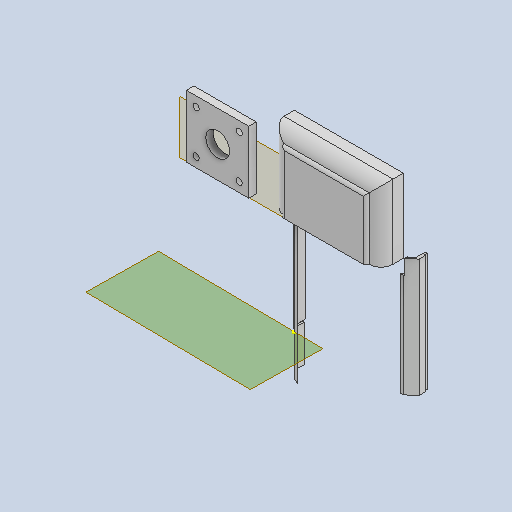
# Autodesk Inventor part: крышка камера
Saved by Autodesk Inventor 2024.2 (Build 282272000, 272)
## iProperties
Created: 2025-10-05
Part Number: крышка камера
Material: Типовые
Document SubType Name: Modeling
Designer: katya_notebook
Density: 1 g/cm^3
Appearance: По умолчанию
Author: katya_notebook
Autodesk Inventor part; units mm, degrees
ref_plane "YZ Plane" through (0, 0, 0) normal (1, 0, 0) x (0, 1, 0)
ref_plane "XZ Plane" through (0, 0, 0) normal (0, 1, 0) x (-1, 0, 0)
ref_plane "XY Plane" through (0, 0, 0) normal (0, 0, 1) x (1, 0, 0)
ref_plane "РабПлоскость1" through (0, 97.1605, 0) normal (0, 0, 1) x (-1, 0, 0)
sketch "Эскиз1" plane through (0, 97.1605, 0) normal (0, 0, 1) x (-1, 0, 0)
  line L0 (53.6991, 17.5343) -> (19.6991, 17.5343) projected
  line L1 (0, -26.68) -> (0, 17.5343)
  line L2 (0, 17.5343) -> (-73.3991, 17.5343)
  line L3 (-73.3991, -26.68) -> (-73.3991, 17.5343)
  line L4 (0, -26.68) -> (0, -32.1685)
  line L5 (-73.3991, -26.68) -> (-73.3991, -32.1685)
  line L6 (-73.3991, -32.1685) -> (0, -32.1685)
  line L7 (-73.3991, 110.6606) -> (-73.3991, 83.6606) projected
  constraints: 12 end point, 2 perpendicular, 1 horizontal, 1 vertical
extrude "Выдавливание1" add sketch "Эскиз1" along normal blind 15
sketch "Эскиз2" plane through (0, 97.1605, 0) normal (0, 0, -1) x (1, 0, 0)
  point P0 (0, 97.1605)
sketch "Эскиз3" plane through (0, 97.1605, 0) normal (0, 0, 1) x (-1, 0, 0)
  circle A0 centre (36.6991, -1.4657) radius 8 projected
  line L0 (53.6991, 17.5343) -> (19.6991, 17.5343) projected
  line L1 (19.6991, -20.4657) -> (53.6991, -20.4657) projected
  line L2 (17.6991, 15.5343) -> (17.6991, -18.4657) projected
  line L3 (55.6991, -18.4657) -> (55.6991, 15.5343) projected
  line L4 (57.6991, 19.5343) -> (15.6991, 19.5343)
  line L5 (15.6991, 19.5343) -> (15.6991, -22.4657)
  line L6 (15.6991, -22.4657) -> (57.6991, -22.4657)
  line L7 (57.6991, -22.4657) -> (57.6991, 19.5343)
  line L8 (57.6991, 19.5343) -> (15.6991, -22.4657) construction
  line L9 (15.6991, 19.5343) -> (57.6991, -22.4657) construction
  point P0 (0, 97.1605)
  dimension "d2" = 42
  dimension "d3" = 42
  constraints: 12 end point, 2 midpoint, 2 parallel, 1 horizontal, 1 perpendicular
  measures "d2" distance of L6.end L5.end
  measures "d3" distance of L4.start L6.end
extrude "Выдавливание2" cut sketch "Эскиз3" along normal blind 15
sketch "Эскиз4" plane through (36.6991, -1.4657, 15) normal (0, 0, 1) x (1, 0, 0)
  circle A0 centre (0, 0) radius 8
  point P0 (-36.6991, 1.4657)
  dimension "d8" = 16
  constraints: 1 centre point
  measures "d8" diameter of A0
extrude "Выдавливание3" cut sketch "Эскиз4" against normal blind 15
sketch "Эскиз5" plane through (0, 97.1605, 15) normal (0, 0, 1) x (-1, 0, 0)
  line L0 (15.6991, 19.5343) -> (57.6991, 19.5343) projected
  line L1 (15.6991, -22.4657) -> (15.6991, 19.5343) projected
  line L2 (15.6991, 19.5343) -> (57.6991, 19.5343)
  line L3 (57.6991, 19.5343) -> (57.6991, -22.4657)
  line L4 (57.6991, -22.4657) -> (15.6991, -22.4657)
  line L5 (15.6991, -22.4657) -> (15.6991, 19.5343)
  circle A0 centre (36.6991, -1.4657) radius 8 projected
  circle A1 centre (36.6991, -1.4657) radius 8
  point P0 (0, 97.1605)
  constraints: 8 end point, 2 parallel, 1 centre point, 1 coincident, 1 concentric, 1 horizontal, 1 perpendicular
extrude "Выдавливание4" add sketch "Эскиз5" against normal blind 5
sketch "Эскиз6" plane through (0, 97.1605, 15) normal (0, 0, 1) x (-1, 0, 0)
  circle A0 centre (4.8591, -20.5207) radius 1.7 projected
  circle A1 centre (68.6491, -20.5207) radius 1.7 projected
  point P0 (0, 97.1605)
extrude "Выдавливание5" cut sketch "Эскиз6" against normal blind 15
ref_plane "РабПлоскость2" through (-83.6534, 0, 27.511) normal (0, -1, 0) x (0.9999139, 0, 0.0131203)
sketch "Эскиз7" plane through (-83.6534, 0, 27.511) normal (0, -1, 0) x (0.9999139, 0, 0.0131203)
  line L0 (79.6013, -33.3861) -> (83.2852, -28.6062) projected
  line L1 (79.5461, -37.5999) -> (79.6013, -33.3861) projected
  line L2 (75.3464, -37.5448) -> (79.5461, -37.5999) projected
  line L3 (83.2852, -28.6062) -> (79.6013, -33.3861)
  line L4 (79.6013, -33.3861) -> (79.5461, -37.5999)
  line L5 (1622.9751, -57.8519) -> (79.5461, -37.5999)
  line L6 (1622.9751, -57.8519) -> (1622.9751, -55.8519)
  line L7 (1622.9751, -55.8519) -> (1621.8385, -55.8519)
  line L8 (1621.8385, -55.8519) -> (1619.8385, -55.8519)
  line L9 (83.2852, -28.6062) -> (85.2851, -28.6324)
  line L10 (156.6781, -29.5692) -> (83.2852, -28.6062) projected
  line L11 (80.8455, -31.8201) -> (80.8455, -55.8519)
  line L12 (80.8455, -55.8519) -> (1619.8385, -55.8519)
  line L13 (80.8455, -31.8201) -> (85.2851, -28.6324)
  line L14 (46.6, -4.8277) -> (46.6, -53.2548)
  line L15 (13.5987, -33.3861) -> (9.9148, -28.6062)
  line L16 (13.6539, -37.5999) -> (13.5987, -33.3861)
  line L17 (9.9148, -28.6062) -> (13.5987, -33.3861)
  line L18 (13.5987, -33.3861) -> (13.6539, -37.5999)
  line L19 (-1529.7751, -57.8519) -> (13.6539, -37.5999)
  line L20 (-1529.7751, -57.8519) -> (-1529.7751, -55.8519)
  line L21 (-1529.7751, -55.8519) -> (-1528.6385, -55.8519)
  line L22 (-1528.6385, -55.8519) -> (-1526.6385, -55.8519)
  line L23 (9.9148, -28.6062) -> (7.9149, -28.6324)
  line L24 (12.3545, -31.8201) -> (12.3545, -55.8519)
  line L25 (12.3545, -55.8519) -> (-1526.6385, -55.8519)
  line L26 (12.3545, -31.8201) -> (7.9149, -28.6324)
  point P0 (87.0301, -15.4429)
  point P1 (85.1096, -24.071)
  point P2 (-1456.642, -15.4429)
  point P3 (1470.5529, -55.8519)
  point P4 (80.8455, -37.617)
  dimension "d13" = 2
  dimension "d14" = 2
  dimension "d15" = 2
  dimension "d16" = 2
  constraints: 46 end point, 10 symmetric about line, 3 vertical, 2 collinear, 2 horizontal, 2 perpendicular, 2 point on line
  measures "d13" distance of L6.end L5.start
  measures "d14" distance of L8.end L7.end
  measures "d15" distance of L0.end L9.end
  measures "d16" distance of L11.start L0.start
ref_plane "РабПлоскость3" through (-3.0009, -24.18, -16.4278) normal (0.7071068, 0.7071068, 0) x (-0.7071068, 0.7071068, 0)
extrude "Выдавливание6" add sketch "Эскиз7" against normal up to surface contours L0 L9 L13 L11 L5 L1 surface through (-3.0009, -24.18, -16.4278) normal (0.7071068, 0.7071068, 0)
ref_plane "РабПлоскость4" through (-83.6534, 0, 27.511) normal (0, -1, 0) x (0.9999139, 0, 0.0131203)
sketch "Эскиз8" plane through (-83.6534, 0, 27.511) normal (0, -1, 0) x (0.9999139, 0, 0.0131203)
  line L0 (6.28, -18.2609) -> (9.8931, -27.6692)
  line L1 (9.8931, -27.6692) -> (11.8779, -27.6692)
  line L2 (156.6781, -29.5692) -> (83.2852, -28.6062) projected
  line L3 (6.28, -9.4429) -> (6.28, -18.2609)
  line L4 (12.3545, -31.8201) -> (7.9149, -28.6324) projected
  line L5 (7.9149, -28.6324) -> (12.3545, -31.8201)
  line L6 (12.3545, -31.8201) -> (12.3545, -55.8519)
  line L7 (-1529.7751, -57.8519) -> (13.6539, -37.5999) projected
  line L8 (-1529.7751, -57.8519) -> (-1529.7751, -55.8519) projected
  line L9 (-1529.7751, -55.8519) -> (-1528.6385, -55.8519) projected
  line L10 (-1529.7751, -57.8519) -> (-1529.7751, -55.8519)
  line L11 (12.3545, -31.8201) -> (12.3545, -55.8519) projected
  line L12 (-1529.7751, -55.8519) -> (12.3545, -55.8519)
  line L13 (-1529.7751, -57.8519) -> (13.6539, -37.5999)
  point P0 (83.2852, -28.6062)
  point P1 (6.28, -15.4429)
  point P2 (6.28, -17.4429)
  point P3 (9.1273, -24.7278)
  constraints: 14 end point, 2 horizontal, 2 vertical, 1 point on line, 7 other
ref_plane "РабПлоскость5" through (73.8991, -26.68, -16.4278) normal (-0.7071068, 0.7071068, 0) x (0, 0, 1)
extrude "Выдавливание7" [suppressed]
fillet "Сопряжение2" radius 8 3 edges at (0, 104.4776, 15) (36.6996, 129.3291, 15) (73.3991, 104.4776, 15)
sketch "Эскиз9" plane through (0, 97.1605, 10) normal (0, 0, -1) x (1, 0, 0)
  circle A0 centre (-36.6991, -1.4657) radius 8 projected
  line L0 (-22.1991, -15.9657) -> (-51.1991, -15.9657)
  line L1 (-51.1991, -15.9657) -> (-51.1991, 13.0343)
  line L2 (-51.1991, 13.0343) -> (-22.1991, 13.0343)
  line L3 (-22.1991, 13.0343) -> (-22.1991, -15.9657)
  line L4 (-22.1991, -15.9657) -> (-51.1991, 13.0343) construction
  line L5 (-51.1991, -15.9657) -> (-22.1991, 13.0343) construction
  circle A1 centre (-51.1991, 13.0343) radius 2.1
  circle A2 centre (-51.1991, -15.9657) radius 2.1
  circle A3 centre (-22.1991, 13.0343) radius 2.1
  circle A4 centre (-22.1991, -15.9657) radius 2.1
  point P0 (0, 97.1605)
  dimension "d23" = 29
  dimension "d24" = 4.2
  constraints: 12 end point, 4 centre point, 4 coincident, 3 equal radius, 2 midpoint, 2 parallel, 2 perpendicular, 1 horizontal
  measures "d23" distance of L1.end L2.end
  measures "d24" diameter of A4
extrude "Выдавливание8" cut sketch "Эскиз9" against normal blind 5 contours A2 L1 L0 | L0 L1 A2 | A4 L3 L0 | L0 L3 A4 | A1 L2 L1 | L1 L2 A1 | A3 L2 L3 | L3 L2 A3
sketch "Эскиз10" plane through (0, 97.1605, 15) normal (0, 0, 1) x (-1, 0, 0)
  line L0 (-8, -24.1685) -> (-65.3991, -24.1685) projected
  line L1 (-8, 17.5343) -> (-8, -24.1685) projected
  line L2 (-65.3991, -24.1685) -> (-65.3991, 17.5343) projected
  line L3 (-8, 17.5343) -> (-65.3991, 17.5343) projected
  point P0 (0, 97.1605)
  constraints: 2 horizontal alignment
extrude "Выдавливание9" add sketch "Эскиз10" along normal blind 2
fillet "Сопряжение3" [suppressed]
fillet "Сопряжение4" radius 2 3 edges at (36.6996, 121.3291, 17) (65.3991, 100.4776, 17) (8, 100.4776, 17)
sketch "Эскиз11" plane through (0, 97.1605, 0) normal (0, 0, -1) x (1, 0, 0)
  spline S0 degree 3 poles (-65.0891, 2.7019) (-65.1607, 2.5849) (-65.2458, 2.4783) (-65.49, 2.2345) (-65.6826, 2.1034) (-66.102, 1.9309) (-66.3287, 1.8893) (-66.7585, 1.8893) (-66.9894, 1.9341) (-67.411, 2.1121) (-67.6019, 2.2451) (-67.8974, 2.5465) (-68.0249, 2.7335) (-68.1958, 3.1474) (-68.2391, 3.3744) (-68.2391, 3.8043) (-68.1958, 4.0313) (-68.0249, 4.4451) (-67.8974, 4.6322) (-67.6019, 4.9335) (-67.411, 5.0665) (-66.9894, 5.2445) (-66.7585, 5.2893) (-66.3287, 5.2893) (-66.102, 5.2477) (-65.6826, 5.0752) (-65.49, 4.9442) (-65.2458, 4.7003) (-65.1607, 4.5937) (-65.0891, 4.4767) knots 0.089167 0.089167 0.089167 0.089167 0.128222 0.128222 0.192735 0.192735 0.257248 0.257248 0.324519 0.324519 0.391791 0.391791 0.456277 0.456277 0.520762 0.520762 0.585248 0.585248 0.649734 0.649734 0.717005 0.717005 0.784277 0.784277 0.84879 0.84879 0.913303 0.913303 0.952358 0.952358 0.952358 0.952358 projected
  arc A0 (-65.0891, 2.7019) -> (-65.0891, 4.4767) centre (-66.5391, 3.5893) ccw projected
  spline S1 degree 3 poles (-4.0891, 4.6354) (-4.0453, 4.6915) (-3.9986, 4.744) (-3.7981, 4.9442) (-3.6057, 5.0751) (-3.1865, 5.2476) (-2.9598, 5.2893) (-2.5302, 5.2893) (-2.2995, 5.2446) (-1.8783, 5.0671) (-1.6875, 4.9344) (-1.3914, 4.6332) (-1.2636, 4.4457) (-1.0923, 4.0313) (-1.0491, 3.8042) (-1.0491, 3.5893) (-1.0491, 3.3744) (-1.0923, 3.1473) (-1.2636, 2.7329) (-1.3914, 2.5454) (-1.6875, 2.2442) (-1.8783, 2.1115) (-2.2995, 1.934) (-2.5302, 1.8893) (-2.9598, 1.8893) (-3.1865, 1.931) (-3.6057, 2.1035) (-3.7981, 2.2344) (-3.9986, 2.4346) (-4.0453, 2.4871) (-4.0891, 2.5432) knots -0.412165 -0.412165 -0.412165 -0.412165 -0.391556 -0.391556 -0.327162 -0.327162 -0.262769 -0.262769 -0.195855 -0.195855 -0.128941 -0.128941 -0.06447 -0.06447 0 0 0 0.06447 0.06447 0.128941 0.128941 0.195855 0.195855 0.262769 0.262769 0.327162 0.327162 0.391556 0.391556 0.412165 0.412165 0.412165 0.412165 projected
  arc A1 (-4.0891, 4.6354) -> (-4.0891, 2.5432) centre (-2.7491, 3.5893) ccw projected
  line L0 (-2.7491, 3.5893) -> (-4.8591, 3.5893)
  circle A2 centre (-4.8591, 3.5893) radius 2.1
  line L1 (-66.5391, 3.5893) -> (-64.4291, 3.5893)
  circle A3 centre (-64.4291, 3.5893) radius 2.1
  point P0 (0, 97.1605)
  dimension "d38" = 2.11
  dimension "d39" = 4.2
  constraints: 4 end point, 3 coincident, 2 centre point, 2 horizontal, 1 collinear, 1 equal radius
  measures "d38" distance of L0.start L0.end
  measures "d39" diameter of A2
extrude "Выдавливание10" cut sketch "Эскиз11" against normal blind 5 contours A0 S0 A3 | S0 A3 L1 A0 | L1 A3 S0 A0 | A1 S1 A2 | S1 A2 L0 A1 | L0 A2 S1 A1
sketch "Эскиз12" plane through (0, 79.6262, 0) normal (0, -1, 0) x (1, 0, 0)
  line L0 (-2.3974, -3.2457) -> (2, 0) projected
  line L1 (2, 0) -> (0, 0) projected
  line L2 (0, 0) -> (-3.6209, -4.8278) projected
  line L3 (10, 17) -> (63.3991, 17) projected
  line L4 (36.6996, 17) -> (36.6996, -97.4622)
  line L5 (78.3462, -9.042) -> (78.3462, -11.042)
  line L6 (78.3462, -11.042) -> (77.1301, -11.042)
  line L7 (77.1301, -11.042) -> (77.1301, -4.8278)
  line L8 (77.1301, -4.8278) -> (71.3991, 0)
  line L9 (71.3991, 0) -> (73.3991, 0)
  line L10 (73.3991, 0) -> (79.1301, -4.8278)
  line L11 (79.1301, -4.8278) -> (79.1301, -9.042)
  line L12 (79.1301, -9.042) -> (78.3462, -9.042)
  line L13 (-3.6209, -4.8278) -> (-3.6209, -9.042) projected
  line L14 (-3.6209, -9.042) -> (-2.3213, -9.042) projected
  line L15 (-2.3213, -9.042) -> (-2.3974, -3.2457) projected
  point P0 (0, 0)
  constraints: 18 end point, 3 symmetric about line, 1 midpoint, 1 vertical
ref_plane "РабПлоскость6" through (-16.7083, 0, -45.6496) normal (0, -1, 0) x (1, 0, 0)
extrude "Выдавливание11" add sketch "Эскиз12" along normal up to surface (79.6262 mm away) contours L5 L6 L7 L8 L9 L10 L11 L12
sketch "Эскиз13" plane through (2, 79.6262, 0) normal (0, -1, 0) x (1, 0, 0)
  line L0 (71.8991, -2.174) -> (69.1444, -2.174)
  line L1 (69.1444, -2.174) -> (69.1444, 0.3398)
  line L2 (69.1444, 0.3398) -> (71.8991, 0.3398)
  line L3 (71.8991, 0.3398) -> (71.8991, -2.174)
  point P0 (-2, 0)
  constraints: 8 end point, 2 parallel, 1 horizontal, 1 perpendicular
extrude "Выдавливание12" cut sketch "Эскиз13" along normal blind 10
sketch "Эскиз14" plane through (0, 97.1605, 0) normal (0, 0, -1) x (1, 0, 0)
  spline S0 degree 3 poles (-6.1991, 4.6354) (-6.1554, 4.6915) (-6.1087, 4.744) (-5.9081, 4.9442) (-5.7158, 5.0751) (-5.2966, 5.2476) (-5.0698, 5.2893) (-4.6402, 5.2893) (-4.4096, 5.2446) (-3.9883, 5.0671) (-3.7975, 4.9344) (-3.5015, 4.6332) (-3.3736, 4.4457) (-3.2024, 4.0313) (-3.1591, 3.8042) (-3.1591, 3.5893) (-3.1591, 3.3744) (-3.2024, 3.1473) (-3.3736, 2.7329) (-3.5015, 2.5454) (-3.7975, 2.2442) (-3.9883, 2.1115) (-4.4096, 1.934) (-4.6402, 1.8893) (-5.0698, 1.8893) (-5.2966, 1.931) (-5.7158, 2.1035) (-5.9081, 2.2344) (-6.1087, 2.4346) (-6.1554, 2.4871) (-6.1991, 2.5432) knots -0.412165 -0.412165 -0.412165 -0.412165 -0.391556 -0.391556 -0.327162 -0.327162 -0.262769 -0.262769 -0.195855 -0.195855 -0.128941 -0.128941 -0.06447 -0.06447 0 0 0 0.06447 0.06447 0.128941 0.128941 0.195855 0.195855 0.262769 0.262769 0.327162 0.327162 0.391556 0.391556 0.412165 0.412165 0.412165 0.412165 projected
  spline S1 degree 3 poles (-67.1991, 2.7019) (-67.2707, 2.5849) (-67.3559, 2.4783) (-67.6001, 2.2345) (-67.7927, 2.1034) (-68.2121, 1.9309) (-68.4388, 1.8893) (-68.8685, 1.8893) (-69.0994, 1.9341) (-69.5211, 2.1121) (-69.712, 2.2451) (-70.0075, 2.5465) (-70.135, 2.7335) (-70.3059, 3.1474) (-70.3491, 3.3744) (-70.3491, 3.8043) (-70.3059, 4.0313) (-70.135, 4.4451) (-70.0075, 4.6322) (-69.712, 4.9335) (-69.5211, 5.0665) (-69.0994, 5.2445) (-68.8685, 5.2893) (-68.4388, 5.2893) (-68.2121, 5.2477) (-67.7927, 5.0752) (-67.6001, 4.9442) (-67.3559, 4.7003) (-67.2707, 4.5937) (-67.1991, 4.4767) knots 0.089167 0.089167 0.089167 0.089167 0.128222 0.128222 0.192735 0.192735 0.257248 0.257248 0.324519 0.324519 0.391791 0.391791 0.456277 0.456277 0.520762 0.520762 0.585248 0.585248 0.649734 0.649734 0.717005 0.717005 0.784277 0.784277 0.84879 0.84879 0.913303 0.913303 0.952358 0.952358 0.952358 0.952358 projected
  arc A0 (-6.1991, 4.6354) -> (-6.1991, 2.5432) centre (-4.8591, 3.5893) ccw projected
  arc A1 (-67.1991, 2.7019) -> (-67.1991, 4.4767) centre (-68.6491, 3.5893) ccw projected
  point P0 (0, 97.1605)
sketch "Эскиз15" plane through (0, 79.6262, 0) normal (0, -1, 0) x (1, 0, 0)
  line L0 (73.3991, 0) -> (73.3991, 7) projected
  arc A0 (73.3991, 7) -> (65.3991, 15) centre (65.3991, 7) ccw projected
  arc A1 (65.3991, 15) -> (63.3991, 17) centre (63.3991, 15) ccw projected
  line L1 (10, 17) -> (63.3991, 17) projected
  arc A2 (10, 17) -> (8, 15) centre (10, 15) ccw projected
  arc A3 (8, 15) -> (0, 7) centre (8, 7) ccw projected
  line L2 (0, 0) -> (0, 7) projected
  line L3 (0, 0) -> (71.3991, 0) projected
  line L4 (71.3991, 0) -> (73.3991, 0) projected
  line L5 (73.3991, 0) -> (0, 0) projected
  line L6 (71.3983, 0) -> (73.3991, 0)
  line L7 (28.6991, 17) -> (44.6991, 17) projected
  line L8 (36.6991, 17) -> (36.6991, -14.9367)
  line L9 (1.9965, 0) -> (-3.7318, -4.8278)
  line L10 (-3.7318, -4.8278) -> (-3.7318, -11.042)
  line L11 (-3.7318, -11.042) -> (-4.9479, -11.042)
  line L12 (-4.9479, -11.042) -> (-4.9479, -9.042)
  line L13 (-4.9479, -9.042) -> (-5.7318, -9.042)
  line L14 (-5.7318, -9.042) -> (-5.7318, -4.8278)
  line L15 (-5.7318, -4.8278) -> (-0.0009, 0)
  line L16 (-0.0009, 0) -> (1.9965, 0)
  point P0 (2, 0)
  constraints: 20 end point, 2 collinear, 1 midpoint, 1 symmetric about line, 1 vertical
ref_plane "РабПлоскость7" through (-14.5982, 0, -45.6496) normal (0, -1, 0) x (1, 0, 0)
extrude "Выдавливание13" add sketch "Эскиз15" along normal up to surface (79.6262 mm away) contours L9 L10 L11 L12 L13 L14 L15 L3
sketch "Эскиз17" plane through (-5.7318, 79.6262, -4.8278) normal (-0.6442744, 0, 0.7647944) x (0.7647944, 0, 0.6442744)
  line L0 (0, 0) -> (0, -79.6262) projected
  line L1 (0, 0) -> (15.6431, 0)
  line L2 (15.6431, 0) -> (15.6431, -5.297)
  line L3 (15.6431, -5.297) -> (0, -5.297)
  line L4 (0, -5.297) -> (0, 0)
  point P0 (7.4941, -79.6262)
  point P1 (0, 26.68)
  constraints: 8 end point, 2 parallel, 1 horizontal, 1 perpendicular
extrude "Выдавливание15" cut sketch "Эскиз17" against normal blind 10
sketch "Эскиз18" plane through (0, 97.1605, 0) normal (0, 0, -1) x (1, 0, 0)
  spline S0 degree 3 poles (67.1991, 94.4586) (67.2707, 94.5756) (67.3559, 94.6822) (67.6001, 94.9261) (67.7927, 95.0571) (68.2121, 95.2296) (68.4388, 95.2712) (68.8685, 95.2712) (69.0994, 95.2264) (69.5211, 95.0484) (69.712, 94.9154) (70.0075, 94.6141) (70.135, 94.427) (70.3059, 94.0132) (70.3491, 93.7862) (70.3491, 93.3563) (70.3059, 93.1293) (70.135, 92.7154) (70.0075, 92.5284) (69.712, 92.227) (69.5211, 92.094) (69.0994, 91.916) (68.8685, 91.8712) (68.4388, 91.8712) (68.2121, 91.9128) (67.7927, 92.0853) (67.6001, 92.2164) (67.3559, 92.4602) (67.2707, 92.5668) (67.1991, 92.6838) knots 0.089167 0.089167 0.089167 0.089167 0.128222 0.128222 0.192735 0.192735 0.257248 0.257248 0.324519 0.324519 0.391791 0.391791 0.456277 0.456277 0.520762 0.520762 0.585248 0.585248 0.649734 0.649734 0.717005 0.717005 0.784277 0.784277 0.84879 0.84879 0.913303 0.913303 0.952358 0.952358 0.952358 0.952358 projected
  arc A0 (67.1991, 94.4586) -> (67.1991, 92.6838) centre (68.6491, 93.5712) ccw projected
  spline S1 degree 3 poles (6.1991, 92.5251) (6.1554, 92.469) (6.1087, 92.4165) (5.9081, 92.2163) (5.7158, 92.0854) (5.2966, 91.9129) (5.0698, 91.8712) (4.6402, 91.8712) (4.4096, 91.9159) (3.9883, 92.0934) (3.7975, 92.2261) (3.5015, 92.5273) (3.3736, 92.7148) (3.2024, 93.1292) (3.1591, 93.3563) (3.1591, 93.5712) (3.1591, 93.7861) (3.2024, 94.0132) (3.3736, 94.4276) (3.5015, 94.6151) (3.7975, 94.9163) (3.9883, 95.049) (4.4096, 95.2266) (4.6402, 95.2712) (5.0698, 95.2712) (5.2966, 95.2295) (5.7158, 95.057) (5.9081, 94.9261) (6.1087, 94.7259) (6.1554, 94.6734) (6.1991, 94.6173) knots -0.412165 -0.412165 -0.412165 -0.412165 -0.391556 -0.391556 -0.327162 -0.327162 -0.262769 -0.262769 -0.195855 -0.195855 -0.128941 -0.128941 -0.06447 -0.06447 0 0 0 0.06447 0.06447 0.128941 0.128941 0.195855 0.195855 0.262769 0.262769 0.327162 0.327162 0.391556 0.391556 0.412165 0.412165 0.412165 0.412165 projected
  arc A1 (6.1991, 92.5251) -> (6.1991, 94.6173) centre (4.8591, 93.5712) ccw projected
  circle A2 centre (-4.8591, 3.5893) radius 2.1 projected
  circle A3 centre (-64.4291, 3.5893) radius 2.1 projected
  circle A4 centre (68.6491, 93.5712) radius 2.1
  point P0 (0, 97.1605)
  dimension "d46" = 4.2
  constraints: 1 centre point, 1 coincident
  measures "d46" diameter of A4
extrude "Выдавливание16" [suppressed]
sketch "Эскиз19" plane through (0, 97.1605, 0) normal (0, 0, -1) x (1, 0, 0)
  circle A0 centre (-64.4291, 3.5893) radius 2.1 projected
  point P0 (0, 97.1605)
extrude "Выдавливание17" [suppressed]
